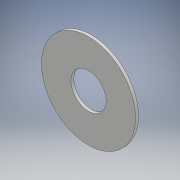
# Autodesk Inventor part: piston_mount_ring_full
Saved by Autodesk Inventor 2018 (Build 220112000, 112)
## iProperties
Created: 2026-05-03
Part Number: piston_mount_ring_full
Material: Generic
Document SubType Name: Modeling
Designer: neo
Density: 1 g/cm^3
Appearance: Default
Author: neo
Autodesk Inventor part; units mm, degrees
ref_plane "YZ Plane" through (0, 0, 0) normal (1, 0, 0) x (0, 1, 0)
ref_plane "XZ Plane" through (0, 0, 0) normal (0, 1, 0) x (-1, 0, 0)
ref_plane "XY Plane" through (0, 0, 0) normal (0, 0, 1) x (1, 0, 0)
sketch "Sketch1" plane through (0, 0, 0) normal (0, 1, 0) x (-1, 0, 0)
  circle A0 centre (0, 0) radius 60
  circle A1 centre (0, 0) radius 160
  dimension "d0" = 320
  dimension "d1" = 100
  dimension "d2" = 120
  constraints: 2 centre point, 2 coincident
  measures "d0" diameter of A1
  measures "d1" radial gap between concentric circles of A1 A0
  measures "d2" diameter of A0
extrude "Extrusion1" add sketch "Sketch1" along normal blind 10
body "Solid1"
